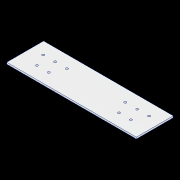
# Autodesk Inventor part: MetalBackArmor
Saved by Autodesk Inventor 2021 (Build 250183000, 183)
## iProperties
Created: 2020-10-24
Part Number: MetalBackArmor
Material: Aluminum 6061
Document SubType Name: Sheet Metal
Designer: Esketitttttt
Density: 2.7 g/cm^3
Sheet Metal Rule: Default
Appearance: Aluminum - Flat
Author: Esketitttttt
Autodesk Inventor part; units mm, degrees
ref_plane "YZ Plane" through (0, 0, 0) normal (1, 0, 0) x (0, 1, 0)
ref_plane "XZ Plane" through (0, 0, 0) normal (0, 1, 0) x (-1, 0, 0)
ref_plane "XY Plane" through (0, 0, 0) normal (0, 0, 1) x (1, 0, 0)
sketch "Sketch1" plane through (0, 0, 0) normal (0, 1, 0) x (-1, 0, 0)
  circle A0 centre (11.26, -23.2833) radius 1.016
  circle A1 centre (94.63, -11.6417) radius 1.016
  circle A2 centre (111.52, -23.2833) radius 1.016
  circle A3 centre (89, -23.2833) radius 1.016
  circle A4 centre (28.15, -11.6417) radius 1.016
  circle A5 centre (22.52, -23.2833) radius 1.016
  circle A6 centre (100.26, -23.2833) radius 1.016
  circle A7 centre (105.89, -11.6417) radius 1.016
  circle A8 centre (33.78, -23.2833) radius 1.016
  circle A9 centre (16.89, -11.6417) radius 1.016
  line L0 (122.78, -34.925) -> (122.78, 0)
  line L1 (0, 0) -> (122.78, 0)
  line L2 (0, 0) -> (0, -34.925)
  line L3 (122.78, -34.925) -> (0, -34.925)
  point P0 (77.74, -31.75)
extrude "Plate1" add sketch "Sketch1" along normal blind 1.5875
sketch "Sketch2" plane through (0, 1.5875, 0) normal (0, 1, 0) x (1, 0, 0)
  circle A0 centre (-16.89, 11.6417) radius 1.016 projected
  circle A1 centre (-33.78, 23.2833) radius 1.016 projected
  circle A2 centre (-105.89, 11.6417) radius 1.016 projected
  circle A3 centre (-100.26, 23.2833) radius 1.016 projected
  circle A4 centre (-22.52, 23.2833) radius 1.016 projected
  circle A5 centre (-28.15, 11.6417) radius 1.016 projected
  circle A6 centre (-89, 23.2833) radius 1.016 projected
  circle A7 centre (-111.52, 23.2833) radius 1.016 projected
  circle A8 centre (-94.63, 11.6417) radius 1.016 projected
  circle A9 centre (-11.26, 23.2833) radius 1.016 projected
  line L0 (-122.78, 34.925) -> (0, 34.925) projected
  line L1 (-122.78, 0) -> (-122.78, 34.925) projected
  line L2 (0, 0) -> (-122.78, 0) projected
  line L3 (0, 34.925) -> (0, 0) projected
hole "Hole1" at (-111.52, 1.5875, -23.2833) at (-105.89, 1.5875, -11.6417) at (-100.26, 1.5875, -23.2833) at (-94.63, 1.5875, -11.6417) at (-89, 1.5875, -23.2833) at (-33.78, 1.5875, -23.2833) at (-28.15, 1.5875, -11.6417) at (-22.52, 1.5875, -23.2833) at (-16.89, 1.5875, -11.6417) at (-11.26, 1.5875, -23.2833) direction (0, -1, 0) diameter 2.1844 depth 1.5875 tip angle 118
equation "\"d6\" = Thickness"
equation "\"d0\" = Thickness"
equation "\"BendRadius\" = Thickness"
equation "\"BendReliefWidth\" = Thickness"
equation "\"BendReliefDepth\" = 0.5 * Thickness"
equation "\"CornerReliefSize\" = 4 * Thickness"
equation "\"MinimumRemnant\" = 2 * Thickness"
equation "\"TransitionRadius\" = BendRadius"
equation "\"JacobiRadiusSize\" = BendRadius"
equation "\"GapSize\" = Thickness"
equation "\"Thickness\" = 1.5875"
body "Solid1"
